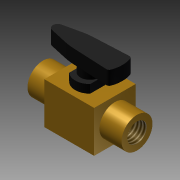
# Autodesk Inventor part: PV609-2
Saved by Autodesk Inventor 2011 (Build 150239000, 239)
## iProperties
Category: Pneumatics
Shininess: 64.0
Length Units: 11272
Angle Units: 11279
Time Units: 11290
Mass Units: 11286
Length Display Precision: 3
Angle Display Precision: 2
Compacted: True
Document SubType Name: Modeling
Created: 2005-01-08
Manufacturer: Standard
Standards Organization: Custom
Vendor: Parker
Project: FIRST
Description: Manual 2 Way Plug Valve
Part Number: PV609-2
Density: 1 g/cm^3
Density: 0.0
Volumn: 0.0
Area: 0.0
PropertySet Name: Model Information
Control State: 0
Master: False
Checked Out: False
Title: Manual 2 Way Plug Valve
Author: Autodesk, Inc.
Autodesk Inventor part; units mm, degrees
ref_plane "YZ Plane" through (0, 0, 0) normal (1, 0, 0) x (0, 1, 0)
ref_plane "XZ Plane" through (0, 0, 0) normal (0, 1, 0) x (-1, 0, 0)
ref_plane "XY Plane" through (0, 0, 0) normal (0, 0, 1) x (1, 0, 0)
sketch "Sketch1" plane through (0, 0, 0) normal (0, 0, 1) x (1, 0, 0)
  line L0 (-11.43, 9.525) -> (11.43, 9.525)
  line L1 (11.43, 9.525) -> (11.43, -9.525)
  line L2 (11.43, -9.525) -> (-11.43, -9.525)
  line L3 (-11.43, -9.525) -> (-11.43, 9.525)
  point P0 (0, 0)
  point P1 (-11.43, 0)
  point P2 (0, 9.525)
  dimension "d0" = 19.05
  dimension "d1" = 22.86
  constraints: 8 end point, 2 midpoint, 2 parallel, 1 horizontal, 1 horizontal alignment, 1 perpendicular, 1 vertical alignment
  measures "d0" distance of L0.end L1.end
  measures "d1" distance of L0.start L0.end
extrude "Extrusion1" add sketch "Sketch1" along normal mid plane 19.05
sketch "Sketch2" plane through (-11.43, -9.525, 9.525) normal (-1, 0, 0) x (0, 0, 1)
  line L0 (0, 0) -> (0, 19.05) projected
  line L1 (-19.05, 19.05) -> (0, 19.05) projected
  line L2 (-19.05, 19.05) -> (-19.05, 0) projected
  line L3 (0, 0) -> (-19.05, 0) projected
  circle A0 centre (-9.525, 9.525) radius 7.112
  point P0 (-9.525, 19.05)
  point P1 (-19.05, 9.525)
  dimension "d4" = 14.224
  constraints: 2 midpoint, 1 centre point, 1 horizontal alignment, 1 vertical alignment
  measures "d4" diameter of A0
extrude "Extrusion2" add sketch "Sketch2" along normal blind 10.16 contours A0
sketch "Sketch3" plane through (11.43, -9.525, 9.525) normal (1, 0, 0) x (0, 0, -1)
  circle A0 centre (9.525, 9.525) radius 7.112
  line L0 (0, 19.05) -> (0, 0) projected
  line L1 (0, 0) -> (19.05, 0) projected
  line L2 (19.05, 0) -> (19.05, 19.05) projected
  line L3 (0, 19.05) -> (19.05, 19.05) projected
  point P0 (9.525, 19.05)
  point P1 (-19.05, 9.525)
  point P2 (0, 9.525)
  point P3 (9.525, 19.05)
  dimension "d7" = 14.224
  constraints: 2 horizontal alignment, 2 midpoint, 2 vertical alignment, 1 centre point
  measures "d7" diameter of A0
extrude "Extrusion3" add sketch "Sketch3" along normal blind 10.16 contours A0
sketch "Sketch4" plane through (-11.43, 9.525, 9.525) normal (0, 1, 0) x (1, 0, 0)
  line L0 (0, 0) -> (22.86, 0) projected
  line L1 (22.86, 0) -> (22.86, 19.05) projected
  line L2 (22.86, 19.05) -> (0, 19.05) projected
  line L3 (0, 19.05) -> (0, 0) projected
  line L4 (16.2654, 14.294) -> (16.2654, 4.756)
  line L5 (6.928, 4.44) -> (6.928, 14.61)
  arc A0 (6.928, 4.44) -> (16.2654, 4.756) centre (11.43, 9.525) ccw
  arc A1 (16.2654, 14.294) -> (6.928, 14.61) centre (11.43, 9.525) ccw
  point P0 (11.43, 19.05)
  point P1 (0, 9.525)
  constraints: 4 end point, 4 point on circle, 2 centre point, 2 midpoint, 1 horizontal alignment, 1 parallel, 1 vertical alignment
extrude "Extrusion4" add sketch "Sketch4" along normal blind 3.81 contours L4 A0 L5 A1
sketch "Sketch5" plane through (-11.43, 13.335, 9.525) normal (0, 1, 0) x (1, 0, 0)
  arc A0 (6.928, 4.44) -> (16.2654, 4.756) centre (11.43, 9.525) ccw projected
  line L0 (16.2654, 14.294) -> (16.2654, 4.756) projected
  arc A1 (16.2654, 14.294) -> (6.928, 14.61) centre (11.43, 9.525) ccw projected
  line L1 (6.928, 4.44) -> (6.928, 14.61) projected
  circle A2 centre (11.43, 9.525) radius 4.3993
  constraints: 1 centre point, 1 coincident
extrude "Extrusion5" add sketch "Sketch5" along normal blind 10.16 contours A2
sketch "Sketch6" plane through (0, 23.495, 0) normal (0, 1, 0) x (1, 0, 0)
  circle A0 centre (0, 0) radius 4.3993 projected
  line L0 (0, 0) -> (16.7523, 0)
  line L1 (0, 0) -> (-17.0377, 0)
  arc A1 (-15.3253, 2.1404) -> (-17.0377, 0) centre (-14.8437, 0) ccw
  line L2 (-15.3253, 2.1404) -> (-7.4316, 3.9165)
  arc A2 (-3.282, 4.4806) -> (-7.4316, 3.9165) centre (-2.0931, -19.81) ccw
  line L3 (-3.282, 4.4806) -> (12.8089, 5.2681)
  arc A3 (14.0126, 4.4806) -> (12.8089, 5.2681) centre (12.8687, 4.0459) ccw
  arc A4 (14.8116, 0) -> (14.0126, 4.4806) centre (2.5491, 0.1246) ccw
  arc A5 (-17.0377, 0) -> (-15.3253, -2.1404) centre (-14.8437, 0) ccw
  line L4 (-15.3253, -2.1404) -> (-7.4316, -3.9165)
  arc A6 (-7.4316, -3.9165) -> (-3.282, -4.4806) centre (-2.0931, 19.81) ccw
  line L5 (-3.282, -4.4806) -> (12.8089, -5.2681)
  arc A7 (12.8089, -5.2681) -> (14.0126, -4.4806) centre (12.8687, -4.0459) ccw
  arc A8 (14.0126, -4.4806) -> (14.8116, 0) centre (2.5491, -0.1246) ccw
  constraints: 16 point on circle, 12 end point, 8 centre point, 8 symmetric about line, 5 tangent, 2 point on line, 1 collinear, 1 horizontal, 6 other
extrude "Extrusion6" add sketch "Sketch6" against normal blind 6.35
sketch "Sketch7" plane through (21.59, 0, 0) normal (1, 0, 0) x (0, 0, -1)
  circle A0 centre (0, 0) radius 4.445
  dimension "d16" = 8.89
  constraints: 1 centre point
  measures "d16" diameter of A0
extrude "Extrusion7" cut sketch "Sketch7" against normal blind 9.525
sketch "Sketch8" plane through (-21.59, 0, 0) normal (-1, 0, 0) x (0, 0, 1)
  circle A0 centre (0, 0) radius 4.445
  dimension "d19" = 8.89
  constraints: 1 centre point
  measures "d19" diameter of A0
extrude "Extrusion8" cut sketch "Sketch8" against normal blind 9.525
sketch "Sketch9" plane through (-12.065, 0, 0) normal (-1, 0, 0) x (0, 0, 1)
  circle A0 centre (0, 0) radius 1.5875
  dimension "d23" = 3.175
  constraints: 1 centre point
  measures "d23" diameter of A0
extrude "Extrusion9" cut sketch "Sketch9" against normal blind 71.4502
thread "Thread1" size "3/8-16 UNC" class "1B" standard "ANSI Unified Screw Threads" full length
thread "Thread2" size "3/8-16 UNC" class "1B" standard "ANSI Unified Screw Threads" full length
sketch "Sketch10" plane through (-11.43, -9.525, 9.525) normal (0, -1, 0) x (1, 0, 0)
  circle A0 centre (11.43, -9.525) radius 4.3993 projected
extrude "Extrusion10" add sketch "Sketch10" along normal blind 1.6002
body "Solid1"
